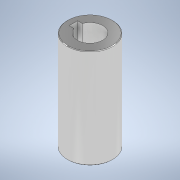
# Autodesk Inventor part: outputshaft nmrv-40
Saved by Autodesk Inventor 2020 (Build 240168000, 168)
## iProperties
Created: 2020-08-01
Part Number: outputshaft nmrv-40
Material: Generic
Document SubType Name: Modeling
Designer: Vikki
Density: 1 g/cm^3
Appearance: Chrome - Polished
Author: Vikki
Autodesk Inventor part; units mm, degrees
ref_plane "YZ Plane" through (0, 0, 0) normal (1, 0, 0) x (0, 1, 0)
ref_plane "XZ Plane" through (0, 0, 0) normal (0, 1, 0) x (-1, 0, 0)
ref_plane "XY Plane" through (0, 0, 0) normal (0, 0, 1) x (1, 0, 0)
sketch "Sketch1" plane through (0, 0, 0) normal (0, 1, 0) x (-1, 0, 0)
  circle A0 centre (0, 0) radius 16
  circle A1 centre (0, 0) radius 9
  line L0 (11.8, 3) -> (11.8, -3)
  line L1 (11.8, 3) -> (8.4853, 3)
  line L2 (11.8, -3) -> (8.4853, -3)
  dimension "d0" = 32
  dimension "d1" = 18
  dimension "d2" = 11.8
  dimension "d3" = 6
  dimension "d4" = 3
  constraints: 6 end point, 2 centre point, 2 coincident, 2 horizontal, 2 point on circle, 1 vertical
  measures "d0" diameter of A0
  measures "d1" diameter of A1
  measures "d2" distance from line of point (0, 0) L0
  measures "d3" distance of L0.start L0.end
  measures "d4" vertical distance of point (0, 0) L0.start
extrude "Extrusion1" add sketch "Sketch1" along normal blind 70
chamfer "Chamfer1" distance 0.4 angle 45 2 edges at (16, 70, 0) (16, 0, 0)
body "Solid1"
